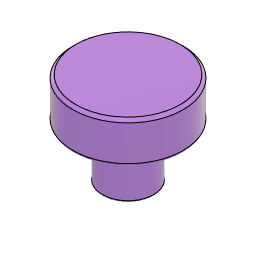
Shutter_Cap _parametric (Autodesk Fusion 360 design; units mm, degrees)
Autodesk Fusion 360 part; units mm, degrees
sketch "Sketch1" plane through (0, 0, 0) normal (0, 1, 0) x (1, 0, 0)
  circle A0 centre (0, 0) radius 1.75
  dimension "d135" = 3.5
  constraint coincident A0.centre origin
  measures "d135" diameter of A0
extrude "Extrude1" add sketch "Sketch1" along normal blind 3.5
sketch "Sketch2" plane through (0, 3.5, 0) normal (0, 1, 0) x (-1, 0, 0)
  circle A0 centre (0, 0) radius 1.75
  circle A1 centre (0, 0) radius 3.75
  dimension "d138" = 7.5
  constraint coincident A0.centre A1.centre
  measures "d138" diameter of A1
extrude "Extrude2" add sketch "Sketch2" along normal blind 2.8 contours A0 | A1
sketch "Sketch3" plane through (0, 0, 0) normal (0, -1, 0) x (1, 0, 0)
  circle A0 centre (0, 0) radius 1.75
  line L0 (1.25, -0.375) -> (-1.25, -0.375)
  line L1 (-1.25, -0.375) -> (-1.25, 0.375)
  line L2 (-1.25, 0.375) -> (1.25, 0.375)
  line L3 (1.25, 0.375) -> (1.25, -0.375)
  line L4 (1.25, -0.375) -> (-1.25, 0.375) construction
  line L5 (-1.25, -0.375) -> (1.25, 0.375) construction
  dimension "d141" = 2.5
  dimension "d142" = 0.75
  constraint horizontal L0
  constraint perpendicular L0 L1
  constraint parallel L0 L2
  constraint parallel L1 L3
  constraint coincident L4 A0.centre
  constraint coincident L5 A0.centre
  constraint coincident A0.centre origin
  measures "d141" distance of L1.end L2.end
  measures "d142" distance of L0.end L1.end
extrude "Extrude3" cut sketch "Sketch3" against normal blind 2 contours L0 L1 L2 L3
fillet "Fillet1" radius 0.2 4 edges at (-1.25, 0, 0) (0, 0, 0.375) (1.25, 0, 0) (0, 0, -0.375)
fillet "Fillet2" radius 0.1 1 edges at (-1.6316, 0, 0.6328)
fillet "Fillet3" radius 0.2 1 edges at (-1.6316, 3.5, 0.6328)
fillet "Fillet4" radius 0.2 1 edges at (3.4962, 3.5, -1.3561)
chamfer "Chamfer1" distance 0.2 angle 45 1 edges at (3.4962, 6.3, -1.3561)
equation "d135 = Shaft_Dia"
equation "d136 = Shaft_Length"
equation "d138 = Head_Dia"
equation "d139 = Head_Thk"
equation "d141 = Slot_Length"
equation "d142 = Slot_Width"
equation "d143 = -Slot_Depth"
equation "Head_Dia = 7.5 mm"
equation "Shaft_Dia = 3.5 mm"
equation "Head_Thk = 2.8 mm"
equation "Shaft_Length = 3.5 mm"
equation "Slot_Depth = 2 mm"
equation "Slot_Width = 0.75 mm"
equation "Slot_Length = 2.5 mm"
named bodies: "Shutter_Cap"
